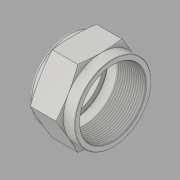
# Autodesk Inventor part: AN818-32D
Saved by Autodesk Inventor 2019 (Build 230136000, 136)
## iProperties
Created: 2018-11-23
Part Number: AN818-32D
Material: Aluminum 2014-T6
Document SubType Name: Modeling
Designer: erics
Density: 2.78927 g/cm^3
Appearance: Satin
Mass: 171.973 g
Surface Area: 231.88 cm^2
Volume: 61.6551 cm^3
Author: erics
Autodesk Inventor part; units mm, degrees
ref_plane "YZ Plane" through (0, 0, 0) normal (1, 0, 0) x (0, 1, 0)
ref_plane "XZ Plane" through (0, 0, 0) normal (0, 1, 0) x (-1, 0, 0)
ref_plane "XY Plane" through (0, 0, 0) normal (0, 0, 1) x (1, 0, 0)
sketch "Sketch1" plane through (0, 0, 0) normal (0, 0, 1) x (1, 0, 0)
  line L0 (2.7686, -36.5125) -> (43.815, -36.5125)
  line L1 (44.196, -36.1315) -> (44.196, -32.131)
  line L2 (43.815, -31.75) -> (7.3152, -31.75)
  line L3 (7.0612, -31.496) -> (7.0612, -27.9019)
  line L4 (6.6802, -27.5209) -> (0.381, -27.5209)
  line L5 (0, -33.7439) -> (0, -27.9019)
  arc A0 (0, -33.7439) -> (2.7686, -36.5125) centre (2.7686, -33.7439) ccw
  line L6 (0.381, -27.5209) -> (0, -27.9019)
  line L7 (6.6802, -27.5209) -> (7.0612, -27.9019)
  line L8 (43.815, -36.5125) -> (44.196, -36.1315)
  line L9 (43.815, -31.75) -> (44.196, -32.131)
  arc A1 (7.0612, -31.496) -> (7.3152, -31.75) centre (7.3152, -31.496) ccw
  line L10 (-5.2446, 0) -> (29.737, 0) projected
  point P0 (0, 0)
  point P1 (0, -36.5125)
  point P2 (44.196, -36.5125)
  point P3 (44.196, -31.75)
  point P4 (7.0612, -31.75)
  point P5 (7.0612, -27.5209)
  point P6 (0, -27.5209)
  dimension "d0" = 27.5209
  dimension "d1" = 36.5125
  dimension "d2" = 44.196
  dimension "d3" = 37.1348
  dimension "d4" = 2.7686
  dimension "d5" = 0.381
  dimension "d6" = 0.381
  dimension "d7" = 0.381
  dimension "d8" = 0.381
  dimension "d9" = 0.381
  dimension "d10" = 0.381
  dimension "d11" = 0.381
  dimension "d12" = 0.381
  dimension "d13" = 0.254
  dimension "d14" = 31.75
  constraints: 20 end point, 12 point on line, 4 perpendicular, 4 point on circle, 4 tangent, 2 centre point, 2 vertical alignment, 1 horizontal, 1 vertical
  measures "d0" distance from line of point (0, 0) L4
  measures "d1" distance from line of point (0, 0) L0
  measures "d2" distance of point (0, -36.513) point (44.196, -36.513)
  measures "d3" distance of point (44.196, -31.75) point (7.061, -31.75)
  measures "d4" radius of A0
  measures "d5" distance of L4.end point (0, -27.521)
  measures "d6" distance of L5.end point (0, -27.521)
  measures "d7" distance of L4.start point (7.061, -27.521)
  measures "d8" distance of L3.end point (7.061, -27.521)
  measures "d9" distance of L0.end point (44.196, -36.513)
  measures "d10" distance of L1.start point (44.196, -36.513)
  measures "d11" distance of L2.start point (44.196, -31.75)
  measures "d12" distance of L1.end point (44.196, -31.75)
  measures "d13" radius of A1
  measures "d14" distance from line of point (0, 0) L2
revolve "Revolution1" add sketch "Sketch1" angle 360 about axis through (-10, 0, 0) along (1, 0, 0)
ref_plane "Work Plane1" through (33.0708, 0, 0) normal (1, 0, 0) x (0, 0, -1)
sketch "Sketch2" plane through (33.0708, 0, 0) normal (1, 0, 0) x (0, 0, -1)
  circle A0 centre (0, 0) radius 31.75 projected
  circle A1 centre (0, 0) radius 36.5125 projected
  line L0 (21.0805, 36.5125) -> (42.161, 0)
  line L1 (42.161, 0) -> (21.0805, -36.5125)
  line L2 (21.0805, -36.5125) -> (-21.0805, -36.5125)
  line L3 (-21.0805, -36.5125) -> (-42.161, 0)
  line L4 (-42.161, 0) -> (-21.0805, 36.5125)
  line L5 (-21.0805, 36.5125) -> (21.0805, 36.5125)
  dimension "d24" = 73.025
  constraints: 12 end point, 1 coincident, 1 horizontal, 13 other
  measures "d24" distance between parallel lines of L2 L5
extrude "Extrusion1" add sketch "Sketch2" against normal blind 27.3812 contours A1 L0 L1 | A1 L5 L0 | L1 L2 A1 | A1 L4 L5 | L2 L3 A1 | A1 L3 L4
sketch "Sketch3" plane through (0, 0, 0) normal (0, 1, 0) x (-1, 0, 0)
  line L0 (-43.815, 36.5125) -> (-33.0708, 36.5125) construction
  line L1 (-33.0708, 21.0805) -> (-33.0708, 42.161) construction
  line L2 (-5.6896, 21.0805) -> (-5.6896, 31.6208) construction
  line L3 (-33.0708, 21.0805) -> (-5.6896, 21.0805) construction
  line L4 (-33.0708, 21.0805) -> (-33.0708, 31.6208) construction
  line L5 (-33.0708, 42.161) -> (-5.6896, 42.161) construction
  line L6 (-5.6896, 36.5125) -> (-2.7686, 36.5125) construction
  line L7 (-33.0708, 36.5125) -> (-31.5573, 42.161)
  line L8 (-5.6896, 36.5125) -> (-7.2031, 42.161)
  line L9 (4.8971, 0) -> (-29.3827, 0) projected
  line L10 (-5.6896, 36.5125) -> (-5.6896, 42.161)
  line L11 (-7.2031, 42.161) -> (-5.6896, 42.161)
  line L12 (-31.5573, 42.161) -> (-33.0708, 42.161)
  line L13 (-33.0708, 36.5125) -> (-33.0708, 42.161)
  line L14 (-33.0708, 31.6208) -> (-33.0708, 42.161) projected
  line L15 (-5.6896, 31.6208) -> (-5.6896, 42.161) projected
  point P0 (0, 0)
  dimension "d19" = 15
  dimension "d25" = 15
  constraints: 12 end point, 2 collinear, 2 point on line, 1 perpendicular, 1 vertical
  measures "d19" angle of L1 L7
  measures "d25" angle of L2 L8
revolve "Revolution2" cut sketch "Sketch3" angle 360 about axis through (-10, 0, 0) along (1, 0, 0)
thread "Thread1" size "2 1/2-12 UN" class "3B" standard "ANSI Unified Screw Threads" length 27.7876
equation "\"d0\" = 0.5 * AN818_A"
equation "\"d1\" = 0.5 * AN818_C"
equation "\"d2\" = AN818_M"
equation "\"d3\" = AN818_L"
equation "\"d4\" = AN818_R"
equation "\"d5\" = AN818_U"
equation "\"d6\" = d5"
equation "\"d7\" = d5"
equation "\"d8\" = d7"
equation "\"d9\" = AN818_N"
equation "\"d10\" = d9"
equation "\"d11\" = d9"
equation "\"d12\" = d11"
equation "\"d14\" = 0.5 * AN818_T"
equation "\"d24\" = AN818_P"
equation "\"d17\" = AN818_J"
equation "\"d22\" = AN818_S"
equation "\"AN818_A\" = 55.0418"
equation "\"AN818_B\" = 11.1252"
equation "\"AN818_C\" = 73.025"
equation "\"AN818_H\" = 63.5"
equation "\"AN818_J\" = 27.3812"
equation "\"AN818_L\" = 37.1348"
equation "\"AN818_M\" = 44.196"
equation "\"AN818_N\" = 0.381"
equation "\"AN818_P\" = 73.025"
equation "\"AN818_Q\" = 21.4376"
equation "\"AN818_R\" = 2.7686"
equation "\"AN818_S\" = 27.7876"
equation "\"AN818_U\" = 0.381"
equation "\"AN818_T\" = 63.5"
equation "\"d16\" = -AN818_B"
equation "\"Tube_OD\" = 50.8"
body "Solid1"
